Rotation Base_v5 (Autodesk Fusion 360 design; units mm, degrees)
Autodesk Fusion 360 part; units mm, degrees
sketch "Sketch2" plane through (0, 0, 0) normal (0, 1, 0) x (1, 0, 0)
  line L0 (0, 0) -> (120, 0) construction
  line L1 (0, 0) -> (-75, 0) construction
  circle A0 centre (-75, 0) radius 3
  circle A1 centre (120, 0) radius 3
  line L2 (-83.0515, 1.5) -> (128.8515, 1.5) construction
  line L3 (-71, 16.5) -> (-79, 16.5)
  line L4 (-79, 16.5) -> (-79, 1.5)
  line L5 (-79, 1.5) -> (-71, 1.5)
  line L6 (-71, 1.5) -> (-71, 16.5)
  line L7 (-71, 16.5) -> (-79, 1.5) construction
  line L8 (-79, 16.5) -> (-71, 1.5) construction
  line L9 (124, 1.5) -> (116, 1.5)
  line L10 (116, 1.5) -> (116, 16.5)
  line L11 (116, 16.5) -> (124, 16.5)
  line L12 (124, 16.5) -> (124, 1.5)
  line L13 (124, 1.5) -> (116, 16.5) construction
  line L14 (116, 1.5) -> (124, 16.5) construction
  point P0 (-75, 9)
  point P1 (120, 9)
  dimension "d3" = 120
  dimension "d4" = 75
  dimension "d5" = 6
  dimension "d6" = 6
  dimension "d7" = 1.5
  dimension "d8" = 8
  dimension "d9" = 15
  dimension "d10" = 9
  dimension "d11" = 8
  dimension "d12" = 15
  dimension "d13" = 9
  constraint coincident L0.start L1.start
  constraint horizontal L0
  constraint parallel L0 L1
  constraint coincident L1.end A0.centre
  constraint coincident L0.end A1.centre
  constraint parallel L0 L2
  constraint horizontal L3
  constraint perpendicular L3 L4
  constraint parallel L3 L5
  constraint parallel L4 L6
  constraint coincident L7 P0
  constraint coincident L8 P0
  constraint horizontal L9
  constraint perpendicular L9 L10
  constraint parallel L9 L11
  constraint parallel L10 L12
  constraint coincident L13 P1
  constraint coincident L14 P1
  measures "d3" distance of L0.start L0.end
  measures "d4" distance of L0.start L1.end
  measures "d5" diameter of A0
  measures "d6" diameter of A1
  measures "d7" distance of L0.start L2
  measures "d8" distance of L4.end L5.end
  measures "d9" distance of L3.end L4.end
  measures "d10" distance of L1.end P0
  measures "d11" distance of L10.end L11.end
  measures "d12" distance of L9.end L10.end
  measures "d13" distance of L0.end P1
revolve "Revolve1" add sketch "Sketch2" angle 360 about axis through (0, 0, 1.75) along (0, 0, 1) contours A0 L3 L4 L5 L6 | A1 L9 L10 L11 L12 makes body 1 at (123.3838, -12.3464, -11.5) makes body 2 at (-78.6074, 7.8659, -11.5)
sketch "Sketch3" plane through (0, 0, -16.5) normal (0, 0, -1) x (1, 0, 0)
  circle A0 centre (0, 0) radius 79
  circle A1 centre (0, 0) radius 71
  line L0 (5, 120) -> (-5, 120)
  line L1 (-5, -120) -> (5, -120)
  line L2 (5, 120) -> (-5, -120) construction
  line L3 (-5, 120) -> (5, -120) construction
  line L4 (-120, -5) -> (-120, 5)
  line L5 (120, 5) -> (120, -5)
  line L6 (120, -5) -> (-120, 5) construction
  line L7 (-120, -5) -> (120, 5) construction
  line L8 (-5, 120) -> (-5, 35)
  line L9 (-5, 0.2083) -> (-5, -0.2083)
  line L10 (-5, -35) -> (-5, -120)
  line L11 (5, -120) -> (5, -35)
  line L12 (120, -5) -> (35, -5)
  line L13 (0.2083, -5) -> (-0.2083, -5)
  line L14 (-35, -5) -> (-120, -5)
  line L15 (-120, 5) -> (-35, 5)
  line L16 (35, 5) -> (120, 5)
  line L17 (5, -0.2083) -> (5, 0.2083)
  line L18 (5, 35) -> (5, 120)
  arc A2 (-35, 5) -> (-5, 35) centre (-35, 35) ccw
  arc A3 (5, 35) -> (35, 5) centre (35, 35) ccw
  arc A4 (35, -5) -> (5, -35) centre (35, -35) ccw
  arc A5 (-5, -35) -> (-35, -5) centre (-35, -35) ccw
  circle A6 centre (0, 0) radius 2
  dimension "d15" = 10
  dimension "d16" = 240
  dimension "d17" = 240
  dimension "d18" = 10
  dimension "d19" = 30
  dimension "d21" = 4
  constraint horizontal L0
  constraint perpendicular L0 L8
  constraint parallel L0 L1
  constraint parallel L8 L11
  constraint coincident L2 A0.centre
  constraint coincident L3 A0.centre
  constraint coincident A0.centre A1.centre
  constraint horizontal L12
  constraint perpendicular L4 L12
  constraint parallel L12 L15
  constraint parallel L4 L5
  constraint coincident L6 A0.centre
  constraint coincident L7 A0.centre
  constraint coincident L6 L9.start
  constraint collinear L8 L9
  constraint coincident L7 L9.end
  constraint collinear L9 L10
  constraint coincident L6 L17.start
  constraint collinear L11 L17
  constraint coincident L3 L13.start
  constraint collinear L12 L13
  constraint coincident L2 L13.end
  constraint collinear L13 L14
  constraint collinear L15 L16
  constraint coincident L7 L17.end
  constraint collinear L17 L18
  constraint tangent L8 A2
  constraint tangent L15 A2
  constraint tangent L18 A3
  constraint tangent L16 A3
  constraint equal A2 A3
  constraint tangent L12 A4
  constraint tangent L11 A4
  constraint equal A2 A4
  constraint tangent L10 A5
  constraint tangent L14 A5
  constraint equal A2 A5
  measures "d15" distance of L1.start L1.end
  measures "d16" distance of L0.end L1.start
  measures "d17" distance of L4.end L5.start
  measures "d18" distance of L4.start L4.end
  measures "d19" radius of A2
  measures "d21" diameter of A6
extrude "Extrude1" add sketch "Sketch3" against normal blind 13 contours A0 A1 L12 L16 | A0 L5 L12 L16 | A0 A1 L8 L18 | A0 L0 L8 L18 | A1 L8 L10 L11 L12 L14 L15 L16 L18 A2 A3 A4 A5 | A0 L1 L10 L11 | A0 A1 L10 L11 | A0 A1 L14 L15 | A0 L4 L14 L15 bodies 1 2
ref_plane "WorkPlane1" through (0, 118, 0) normal (0, 1, 0) x (0, 0, 1)
sketch "Sketch4" plane through (0, 118, 0) normal (0, 1, 0) x (1, 0, 0)
  line L0 (-30.23, 16.5) -> (30.23, 16.5)
  line L1 (30.23, 16.5) -> (30.23, 5.5609)
  line L2 (30.23, 5.5609) -> (-30.23, 5.5609)
  line L3 (-30.23, 5.5609) -> (-30.23, 16.5)
  line L4 (-30.23, 16.5) -> (30.23, 5.5609) construction
  line L5 (30.23, 16.5) -> (-30.23, 5.5609) construction
  circle A0 centre (25, 11.0304) radius 1.5
  circle A1 centre (-25, 11.0304) radius 1.5
  point P0 (0, 11.0304)
  dimension "d25" = 3
  dimension "d26" = 25
  dimension "d27" = 3
  dimension "d28" = 25
  constraint horizontal L0
  constraint perpendicular L0 L1
  constraint parallel L0 L2
  constraint parallel L1 L3
  constraint coincident L4 P0
  constraint coincident L5 P0
  constraint collinear L0
  measures "d25" diameter of A0
  measures "d26" distance of P0 A0.centre
  measures "d27" diameter of A1
  measures "d28" distance of P0 A1.centre
extrude "Extrude2" add sketch "Sketch4" along normal blind 23 contours L0 L1 L2 L3 | A0 | A1 bodies 1
extrude "Extrude4" add 1 faces at (0, 135.3333, -5.5609) along direction (0, 0, 1) up to surface (4.0609 mm away) on bodies 1 bodies 1
extrude "Extrude5" add 1 faces at (10.0767, 141, -11.5) along direction (0, 1, 0) blind 45 on bodies 1 bodies 1
sketch "Sketch5" plane through (0, 0, -1.5) normal (0, 0, 1) x (-1, 0, 0)
  arc A0 (30.23, -120.2587) -> (-30.23, -120.2587) centre (0, 0) ccw
  line L0 (-30.23, -120.2587) -> (-30.23, -186)
  line L1 (-30.23, -186) -> (30.23, -186)
  line L2 (30.23, -186) -> (30.23, -120.2587)
  circle A1 centre (0, 0) radius 122.5981
  line L3 (1.4915, -167.7202) -> (1.5, -171.9933)
  line L4 (-1.5, -167.8793) -> (-1.5, -171.9963)
  arc A2 (1.4963, -170.1059) -> (1.4958, -169.8882) centre (0, -170) ccw
  arc A3 (1.4922, -168.0325) -> (-1.5, -167.8793) centre (0, -167.8793) ccw
  arc A4 (-1.5, -171.9963) -> (1.5, -171.9933) centre (0, -171.9963) ccw
  dimension "d37" = 60.4599
  dimension "d38" = 3
  dimension "d39" = 3
  dimension "d40" = 170
  dimension "d41" = 3
  constraint coincident L3.start A3
  constraint tangent L3 A4
  constraint tangent L4 A4
  constraint vertical L4
  constraint coincident L3 A2.end
  constraint coincident L3 A3.start
  constraint coincident L3 A2.start
  measures "d37" distance of L0 L2
  measures "d38" diameter of A3
  measures "d39" diameter of A2
  measures "d40" distance of A0.centre A2.centre
  measures "d41" diameter of A4
extrude "Extrude6" cut sketch "Sketch5" against normal blind 21 contours L3 L4 A3 A4 bodies 1
sketch "Sketch6" plane through (0, 0, -1.5) normal (0, 0, 1) x (-1, 0, 0)
  line L0 (-1.5, -171.9963) -> (-1.5, -167.8793)
  arc A0 (1.4915, -167.7202) -> (-1.5, -167.8793) centre (0, -167.8793) ccw
  line L1 (1.4915, -167.7202) -> (1.5, -171.9933)
  arc A1 (-1.5, -171.9963) -> (1.5, -171.9933) centre (0, -171.9963) ccw
  arc A2 (30.23, -120.2587) -> (-30.23, -120.2587) centre (0, 0) ccw
  line L2 (-30.23, -120.2587) -> (-30.23, -186)
  line L3 (-30.23, -186) -> (30.23, -186)
  line L4 (30.23, -186) -> (30.23, -120.2587)
  circle A3 centre (0, 0) radius 122.5981
  line L5 (-25.23, -151) -> (-15.23, -151)
  line L6 (-15.23, -151) -> (-15.23, -181)
  line L7 (-15.23, -181) -> (-25.23, -181)
  line L8 (-25.23, -181) -> (-25.23, -151)
  line L9 (15.23, -151) -> (25.23, -151)
  line L10 (25.23, -151) -> (25.23, -181)
  line L11 (25.23, -181) -> (15.23, -181)
  line L12 (15.23, -181) -> (15.23, -151)
  dimension "d44" = 10
  dimension "d45" = 30
  dimension "d46" = 5
  dimension "d47" = 5
  dimension "d48" = 10
  dimension "d49" = 30
  dimension "d50" = 5
  dimension "d51" = 5
  constraint horizontal L5
  constraint vertical L6
  constraint horizontal L7
  constraint vertical L8
  constraint horizontal L9
  constraint vertical L10
  constraint horizontal L11
  constraint vertical L12
  measures "d44" distance of L5.start L5.end
  measures "d45" distance of L5.end L6.end
  measures "d46" distance of L3 L7
  measures "d47" distance of L2 L8
  measures "d48" distance of L9.start L9.end
  measures "d49" distance of L9.start L11.end
  measures "d50" distance of L3 L11
  measures "d51" distance of L4 L10
extrude "Extrude7" cut sketch "Sketch6" against normal blind 17 contours L5 L6 L7 L8 | L9 L10 L11 L12 bodies 1
fillet "Fillet1" radius 50 2 edges at (30.23, 120.2587, -9) (-30.23, 120.2587, -9) on bodies 1
sketch "Sketch8" plane through (0, 0, -16.5) normal (0, 0, -1) x (1, 0, 0)
  line L0 (-25.23, -181) -> (-25.23, -151)
  line L1 (-25.23, -151) -> (-15.23, -151)
  line L2 (-15.23, -151) -> (-15.23, -181)
  line L3 (-15.23, -181) -> (-25.23, -181)
  line L4 (15.23, -181) -> (15.23, -151)
  line L5 (15.23, -151) -> (25.23, -151)
  line L6 (25.23, -151) -> (25.23, -181)
  line L7 (25.23, -181) -> (15.23, -181)
  line L8 (1.5, -167.8793) -> (1.5, -171.9963)
  arc A0 (-1.5, -171.9933) -> (1.5, -171.9963) centre (0, -171.9963) ccw
  line L9 (-1.5, -171.9933) -> (-1.4915, -167.7202)
  arc A1 (1.5, -167.8793) -> (-1.4915, -167.7202) centre (0, -167.8793) ccw
  line L10 (-30.23, -154.3993) -> (-30.23, -186)
  line L11 (-30.23, -186) -> (30.23, -186)
  line L12 (30.23, -186) -> (30.23, -154.3993)
  arc A2 (57.1754, -110.0317) -> (30.23, -154.3993) centre (80.23, -154.3993) ccw
  arc A3 (57.1754, -110.0317) -> (-57.1754, -110.0317) centre (0, 0) ccw
  arc A4 (-30.23, -154.3993) -> (-57.1754, -110.0317) centre (-80.23, -154.3993) ccw
  arc A5 (5, -115.8922) -> (115.8922, -5) centre (0, 0) ccw
  line L13 (5, -115.8922) -> (5, -78.8416)
  arc A6 (5, -78.8416) -> (78.8416, -5) centre (0, 0) ccw
  line L14 (78.8416, -5) -> (115.8922, -5)
  line L15 (115.8922, 5) -> (78.8416, 5)
  arc A7 (78.8416, 5) -> (5, 78.8416) centre (0, 0) ccw
  line L16 (5, 78.8416) -> (5, 115.8922)
  arc A8 (115.8922, 5) -> (5, 115.8922) centre (0, 0) ccw
  line L17 (-5, 115.8922) -> (-5, 78.8416)
  arc A9 (-5, 78.8416) -> (-78.8416, 5) centre (0, 0) ccw
  line L18 (-78.8416, 5) -> (-115.8922, 5)
  arc A10 (-5, 115.8922) -> (-115.8922, 5) centre (0, 0) ccw
  line L19 (-70.8237, -5) -> (-35, -5)
  arc A11 (-5, -35) -> (-35, -5) centre (-35, -35) ccw
  line L20 (-5, -35) -> (-5, -70.8237)
  arc A12 (-70.8237, -5) -> (-5, -70.8237) centre (0, 0) ccw
  circle A13 centre (0, 0) radius 2
  line L21 (-5, 70.8237) -> (-5, 35)
  arc A14 (-35, 5) -> (-5, 35) centre (-35, 35) ccw
  line L22 (-35, 5) -> (-70.8237, 5)
  arc A15 (-5, 70.8237) -> (-70.8237, 5) centre (0, 0) ccw
  line L23 (70.8237, 5) -> (35, 5)
  arc A16 (5, 35) -> (35, 5) centre (35, 35) ccw
  line L24 (5, 35) -> (5, 70.8237)
  arc A17 (70.8237, 5) -> (5, 70.8237) centre (0, 0) ccw
  arc A18 (5, -70.8237) -> (70.8237, -5) centre (0, 0) ccw
  line L25 (5, -70.8237) -> (5, -35)
  arc A19 (35, -5) -> (5, -35) centre (35, -35) ccw
  line L26 (35, -5) -> (70.8237, -5)
  line L27 (-115.8922, -5) -> (-78.8416, -5)
  arc A20 (-78.8416, -5) -> (-5, -78.8416) centre (0, 0) ccw
  line L28 (-5, -78.8416) -> (-5, -115.8922)
  arc A21 (-115.8922, -5) -> (-5, -115.8922) centre (0, 0) ccw
  line L29 (3.5, -167.8793) -> (3.5, -171.9963)
  arc A22 (-3.5, -171.9894) -> (3.5, -171.9963) centre (0, -171.9963) ccw
  line L30 (-3.5, -171.9894) -> (-3.4914, -167.6336)
  arc A23 (3.5, -167.8793) -> (-3.4914, -167.6336) centre (0, -167.8793) ccw
  dimension "d66" = 2
extrude "Extrude8" cut sketch "Sketch8" against normal blind 3 contours L29 A22 L30 A23 bodies 1
sketch "Sketch9" plane through (0, 0, -1.5) normal (0, 0, 1) x (-1, 0, 0)
  line L0 (25.23, -151) -> (25.23, -181)
  line L1 (25.23, -181) -> (15.23, -181)
  line L2 (15.23, -181) -> (15.23, -151)
  line L3 (15.23, -151) -> (25.23, -151)
  line L4 (-15.23, -151) -> (-15.23, -181)
  line L5 (-15.23, -181) -> (-25.23, -181)
  line L6 (-25.23, -181) -> (-25.23, -151)
  line L7 (-25.23, -151) -> (-15.23, -151)
  line L8 (-1.5, -171.9963) -> (-1.5, -167.8793)
  arc A0 (1.4915, -167.7202) -> (-1.5, -167.8793) centre (0, -167.8793) ccw
  line L9 (1.4915, -167.7202) -> (1.5, -171.9933)
  arc A1 (-1.5, -171.9963) -> (1.5, -171.9933) centre (0, -171.9963) ccw
  arc A2 (57.1754, -110.0317) -> (-57.1754, -110.0317) centre (0, 0) ccw
  arc A3 (-30.23, -154.3993) -> (-57.1754, -110.0317) centre (-80.23, -154.3993) ccw
  line L10 (-30.23, -154.3993) -> (-30.23, -186)
  line L11 (-30.23, -186) -> (30.23, -186)
  line L12 (30.23, -186) -> (30.23, -154.3993)
  arc A4 (57.1754, -110.0317) -> (30.23, -154.3993) centre (80.23, -154.3993) ccw
  circle A5 centre (0, 0) radius 122.5981
  arc A6 (11.491, -167.4236) -> (-11.5, -167.8793) centre (0, -167.8793) ccw
  line L13 (-11.5, -171.9963) -> (-11.5, -167.8793)
  arc A7 (-11.5, -171.9963) -> (11.5, -171.9735) centre (0, -171.9963) ccw
  line L14 (11.491, -167.4236) -> (11.5, -171.9735)
  dimension "d69" = 10
extrude "Extrude9" cut sketch "Sketch9" against normal blind 3.25 contours A6 L13 A7 L14 bodies 1
sketch "Sketch10" plane through (0, 0, -3.5) normal (0, 0, 1) x (-1, 0, 0)
  circle A0 centre (0, 0) radius 2
  arc A1 (-70.8237, 5) -> (-70.8237, -5) centre (0, 0) ccw
  line L0 (-70.8237, -5) -> (-35, -5)
  arc A2 (-5, -35) -> (-35, -5) centre (-35, -35) ccw
  line L1 (-5, -35) -> (-5, -70.8237)
  arc A3 (-5, -70.8237) -> (5, -70.8237) centre (0, 0) ccw
  line L2 (5, -70.8237) -> (5, -35)
  arc A4 (35, -5) -> (5, -35) centre (35, -35) ccw
  line L3 (35, -5) -> (70.8237, -5)
  arc A5 (70.8237, -5) -> (70.8237, 5) centre (0, 0) ccw
  line L4 (70.8237, 5) -> (35, 5)
  arc A6 (5, 35) -> (35, 5) centre (35, 35) ccw
  line L5 (5, 35) -> (5, 70.8237)
  arc A7 (5, 70.8237) -> (-5, 70.8237) centre (0, 0) ccw
  line L6 (-5, 70.8237) -> (-5, 35)
  arc A8 (-35, 5) -> (-5, 35) centre (-35, 35) ccw
  line L7 (-35, 5) -> (-70.8237, 5)
  circle A9 centre (0, 40) radius 2
  circle A10 centre (0, 100) radius 2
  circle A11 centre (0, 100) radius 4
  circle A12 centre (0, 40) radius 4
  dimension "d72" = 4
  dimension "d73" = 4
  dimension "d74" = 40
  dimension "d75" = 100
  dimension "d78" = 8
  dimension "d79" = 8
  constraint concentric A10 A11
  constraint concentric A9 A12
  measures "d72" diameter of A9
  measures "d73" diameter of A10
  measures "d74" distance of A0.centre A9.centre
  measures "d75" distance of A0.centre A10.centre
  measures "d78" diameter of A11
  measures "d79" diameter of A12
extrude "Extrude10" cut sketch "Sketch10" against normal blind 28 contours A9 | A10 bodies 1
extrude "Extrude11" cut sketch "Sketch10" against normal blind 4 contours A11 | A12 bodies 1
pattern_circular "C-Pattern1" count 4 over 360 about axis through (0, 0, 1.75) along (0, 0, 1) of "Extrude10", "Extrude11"
sketch "Sketch11" plane through (30.23, 0, 0) normal (1, 0, 0) x (0, 1, 0)
  line L0 (154.3993, -1.5) -> (154.3993, -16.5)
  line L1 (154.3993, -16.5) -> (186, -16.5)
  line L2 (186, -16.5) -> (186, -1.5)
  line L3 (186, -1.5) -> (154.3993, -1.5)
  line L4 (160.9995, -7.0039) -> (175.9995, -7)
  line L5 (161.0005, -11.0039) -> (176.0005, -11)
  arc A0 (160.9995, -7.0039) -> (161.0005, -11.0039) centre (161, -9.0039) ccw
  arc A1 (176.0005, -11) -> (175.9995, -7) centre (176, -9) ccw
  dimension "d84" = 4
  dimension "d85" = 4
  dimension "d86" = 10
  dimension "d87" = 15
  constraint tangent L4 A1
  constraint tangent L4 A0
  constraint tangent L5 A1
  constraint tangent L5 A0
  measures "d84" diameter of A1
  measures "d85" diameter of A0
  measures "d86" distance of L2 A1.centre
  measures "d87" distance of A1.centre A0.centre
extrude "Extrude12" cut sketch "Sketch11" against normal blind 7 contours L4 L5 A0 A1 bodies 1
mirror "Mirror1" about plane through (0, 0, 0) normal (1, 0, 0) of "Extrude12"
sketch "Sketch12" plane through (0, 0, -16.5) normal (0, 0, -1) x (1, 0, 0)
  circle A0 centre (-40, 0) radius 2
  circle A1 centre (-100, 0) radius 2
  circle A2 centre (0, -40) radius 2
  circle A3 centre (0, -100) radius 2
  circle A4 centre (40, 0) radius 2
  circle A5 centre (100, 0) radius 2
  circle A6 centre (0, 40) radius 2
  circle A7 centre (0, 100) radius 2
  line L0 (3.5, -167.8793) -> (3.5, -171.9963)
  arc A8 (-3.5, -171.9894) -> (3.5, -171.9963) centre (0, -171.9963) ccw
  line L1 (-3.5, -171.9894) -> (-3.4914, -167.6336)
  arc A9 (3.5, -167.8793) -> (-3.4914, -167.6336) centre (0, -167.8793) ccw
  line L2 (-25.23, -181) -> (-25.23, -151)
  line L3 (-25.23, -151) -> (-15.23, -151)
  line L4 (-15.23, -151) -> (-15.23, -181)
  line L5 (-15.23, -181) -> (-25.23, -181)
  line L6 (15.23, -181) -> (15.23, -151)
  line L7 (15.23, -151) -> (25.23, -151)
  line L8 (25.23, -151) -> (25.23, -181)
  line L9 (25.23, -181) -> (15.23, -181)
  line L10 (-30.23, -154.3993) -> (-30.23, -186)
  line L11 (-30.23, -186) -> (30.23, -186)
  line L12 (30.23, -186) -> (30.23, -154.3993)
  arc A10 (57.1754, -110.0317) -> (30.23, -154.3993) centre (80.23, -154.3993) ccw
  arc A11 (57.1754, -110.0317) -> (-57.1754, -110.0317) centre (0, 0) ccw
  arc A12 (-30.23, -154.3993) -> (-57.1754, -110.0317) centre (-80.23, -154.3993) ccw
  arc A13 (5, -115.8922) -> (115.8922, -5) centre (0, 0) ccw
  line L13 (5, -115.8922) -> (5, -78.8416)
  arc A14 (5, -78.8416) -> (78.8416, -5) centre (0, 0) ccw
  line L14 (78.8416, -5) -> (115.8922, -5)
  line L15 (115.8922, 5) -> (78.8416, 5)
  arc A15 (78.8416, 5) -> (5, 78.8416) centre (0, 0) ccw
  line L16 (5, 78.8416) -> (5, 115.8922)
  arc A16 (115.8922, 5) -> (5, 115.8922) centre (0, 0) ccw
  line L17 (-5, 115.8922) -> (-5, 78.8416)
  arc A17 (-5, 78.8416) -> (-78.8416, 5) centre (0, 0) ccw
  line L18 (-78.8416, 5) -> (-115.8922, 5)
  arc A18 (-5, 115.8922) -> (-115.8922, 5) centre (0, 0) ccw
  line L19 (-70.8237, -5) -> (-35, -5)
  arc A19 (-5, -35) -> (-35, -5) centre (-35, -35) ccw
  line L20 (-5, -35) -> (-5, -70.8237)
  arc A20 (-70.8237, -5) -> (-5, -70.8237) centre (0, 0) ccw
  circle A21 centre (0, 0) radius 2
  line L21 (-5, 70.8237) -> (-5, 35)
  arc A22 (-35, 5) -> (-5, 35) centre (-35, 35) ccw
  line L22 (-35, 5) -> (-70.8237, 5)
  arc A23 (-5, 70.8237) -> (-70.8237, 5) centre (0, 0) ccw
  line L23 (70.8237, 5) -> (35, 5)
  arc A24 (5, 35) -> (35, 5) centre (35, 35) ccw
  line L24 (5, 35) -> (5, 70.8237)
  arc A25 (70.8237, 5) -> (5, 70.8237) centre (0, 0) ccw
  arc A26 (5, -70.8237) -> (70.8237, -5) centre (0, 0) ccw
  line L25 (5, -70.8237) -> (5, -35)
  arc A27 (35, -5) -> (5, -35) centre (35, -35) ccw
  line L26 (35, -5) -> (70.8237, -5)
  line L27 (-115.8922, -5) -> (-78.8416, -5)
  arc A28 (-78.8416, -5) -> (-5, -78.8416) centre (0, 0) ccw
  line L28 (-5, -78.8416) -> (-5, -115.8922)
  arc A29 (-115.8922, -5) -> (-5, -115.8922) centre (0, 0) ccw
  line L29 (4.7177, -0.8404) -> (3.0867, 3.6655)
  line L30 (3.0867, 3.6655) -> (-1.631, 4.5059)
  line L31 (-1.631, 4.5059) -> (-4.7177, 0.8404)
  line L32 (-4.7177, 0.8404) -> (-3.0867, -3.6655)
  line L33 (-3.0867, -3.6655) -> (1.631, -4.5059)
  line L34 (1.631, -4.5059) -> (4.7177, -0.8404)
  dimension "d94" = 4.15
  constraint coincident A11.centre A13.centre
  measures "d94" distance of A11.centre L34
extrude "Extrude14" cut sketch "Sketch12" against normal blind 4 contours L29 L30 L31 L32 L33 L34 bodies 1
equation "d3 = ( 240 / 2 ) * 1 mm"
equation "d4 = ( 150 / 2 ) * 1 mm"
equation "d9 = d12"
equation "d10 = d9 / 2 + 1.5 mm"
equation "d13 = d12 / 2 + 1.5 mm"
equation "d17 = d16"
equation "d18 = d15"
equation "d22 = -d12 + 2 mm"
equation "d48 = d44"
equation "d49 = d45"
equation "d50 = d46"
equation "d51 = d47"
equation "d73 = d72"
equation "d78 = d79"
equation "d94 = ( 8.3 / 2 ) * 1 mm"
